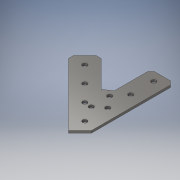
# Autodesk Inventor part: 1in 60deg bracket for alu extrusion
Saved by Autodesk Inventor 2017 (Build 210142000, 142)
## iProperties
Created: 2016-10-02
Part Number: 1in 60deg bracket for alu extrusion
Material: Steel, Alloy
Document SubType Name: Modeling
Designer: Aditya
Density: 7.73 g/cm^3
Appearance: Semi-Polished
Author: Aditya
Autodesk Inventor part; units mm, degrees
ref_plane "YZ Plane" through (0, 0, 0) normal (1, 0, 0) x (0, 1, 0)
ref_plane "XZ Plane" through (0, 0, 0) normal (0, 1, 0) x (-1, 0, 0)
ref_plane "XY Plane" through (0, 0, 0) normal (0, 0, 1) x (1, 0, 0)
sketch "Sketch1" plane through (0, 0, 0) normal (0, 1, 0) x (-1, 0, 0)
  line L0 (0, 0) -> (12.5724, 12.5724)
  line L1 (0, 0) -> (17.78, 0) construction
  line L2 (25.4, -50.8) -> (34.125, -44.9013)
  circle A0 centre (66.4539, -59.2697) radius 2.54
  circle A1 centre (48.4934, -41.3092) radius 2.54
  circle A2 centre (30.5329, -23.3487) radius 2.54
  circle A3 centre (12.5724, -5.3882) radius 2.54
  circle A4 centre (12.5724, -30.7882) radius 2.54
  circle A5 centre (12.5724, -56.1882) radius 2.54
  circle A6 centre (12.5724, -81.5882) radius 2.54
  circle A7 centre (22.86, -43.18) radius 2.54
  circle A8 centre (22.86, -22.86) radius 2.54
  line L3 (81.7203, -56.5756) -> (81.7203, -61.9638)
  line L4 (69.148, -74.5361) -> (63.7598, -74.5361)
  line L5 (21.59, -91.44) -> (25.4, -87.63)
  line L6 (0, -87.63) -> (3.81, -91.44)
  line L7 (81.7203, -61.9638) -> (69.148, -74.5361)
  line L8 (81.7203, -56.5756) -> (12.5724, 12.5724)
  line L9 (0, 0) -> (0, -87.63)
  line L10 (3.81, -91.44) -> (21.59, -91.44)
  line L11 (25.4, -87.63) -> (25.4, -50.8)
  line L12 (34.125, -44.9013) -> (63.7598, -74.5361)
  dimension "d3" = 17.78
  dimension "d4" = 45
  constraints: 26 end point, 9 centre point, 3 perpendicular, 2 horizontal, 2 vertical, 1 equal length, 1 parallel
  measures "d3" distance of L0.start L0.end
  measures "d4" angle of L1 L0
extrude "Extrusion1" add sketch "Sketch1" along normal blind 2.54
body "Solid1"
